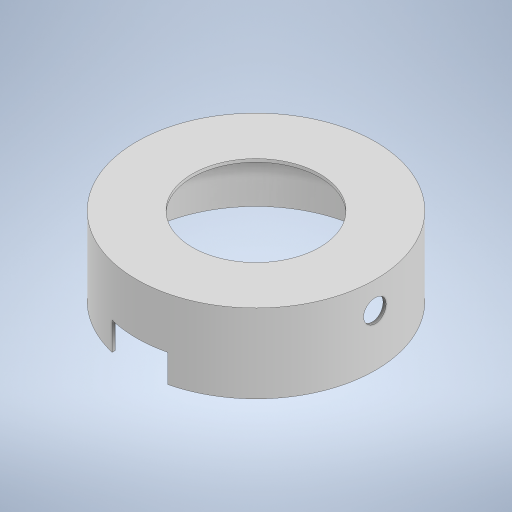
# Autodesk Inventor part: Diaphragm_lock
Saved by Autodesk Inventor 2023 (Build 270158000, 158)
## iProperties
Created: 2023-02-27
Part Number: Diaphragm_lock
Material: Generic
Document SubType Name: Modeling
Designer: maste
Density: 1 g/cm^3
Appearance: Default
Author: maste
Autodesk Inventor part; units mm, degrees
ref_plane "YZ Plane" through (0, 0, 0) normal (1, 0, 0) x (0, 1, 0)
ref_plane "XZ Plane" through (0, 0, 0) normal (0, 1, 0) x (-1, 0, 0)
ref_plane "XY Plane" through (0, 0, 0) normal (0, 0, 1) x (1, 0, 0)
sketch "Sketch1" plane through (0, 0, 0) normal (0, 0, 1) x (1, 0, 0)
  circle A0 centre (0, 0) radius 30
  dimension "d0" = 60
  constraints: 1 centre point, 1 coincident
  measures "d0" diameter of A0
extrude "Initial Cylinder" add sketch "Sketch1" along normal blind 4.78
sketch "Sketch2" plane through (0, 0, 4.78) normal (0, 0, 1) x (1, 0, 0)
  circle A0 centre (0, 0) radius 16
  dimension "d3" = 32
  constraints: 1 centre point, 1 coincident
  measures "d3" diameter of A0
extrude "Through-hole" cut sketch "Sketch2" against normal blind 548
sketch "Sketch3" plane through (0, 0, 4.78) normal (0, 0, 1) x (1, 0, 0)
  circle A0 centre (0, 0) radius 29.25
  dimension "d6" = 58.5
  constraints: 1 centre point, 1 coincident
  measures "d6" diameter of A0
extrude "snug ring fit" cut sketch "Sketch3" against normal blind 4
sketch "Sketch5" plane through (0, 0, 0) normal (0, 1, 0) x (-1, 0, 0)
  line L0 (30, 4.78) -> (-30, 4.78) projected
  line L1 (30, 0) -> (-30, 0) projected
  point P0 (0, 0)
  dimension "d16" = 4.78
  measures "d16" distance between parallel lines of L0 L1
sketch "Sketch6" plane through (0, 0, 0.78) normal (0, 0, 1) x (1, 0, 0)
  circle A0 centre (0, 0) radius 17.65
  dimension "d17" = 35.3
  constraints: 1 centre point, 1 coincident
  measures "d17" diameter of A0
extrude "Piezo Puzzle indent" cut sketch "Sketch6" against normal blind 0.5
sketch "Sketch7" plane through (0, 0, 0) normal (0, 0, -1) x (-1, 0, 0)
  circle A0 centre (0, 0) radius 16 projected
  circle A1 centre (0, 0) radius 30 projected
extrude "Extra forward thickness" add sketch "Sketch7" along normal blind 1
sketch "Sketch8" plane through (0, 0, 0.28) normal (0, 0, 1) x (1, 0, 0)
  circle A0 centre (0, 0) radius 16 projected
  circle A1 centre (0, 0) radius 17.65 projected
  circle A2 centre (0, 0) radius 17.75
  dimension "d26" = 35.5
  constraints: 1 centre point, 1 coincident
  measures "d26" diameter of A2
extrude "Piezo accomodation for EFT^" cut sketch "Sketch8" along normal mid plane 1 contours A0 | A1 | A2
sketch "Sketch9" plane through (0, 0, 4.78) normal (0, 0, 1) x (1, 0, 0)
  circle A0 centre (0, 0) radius 29.25 projected
  circle A1 centre (0, 0) radius 30 projected
extrude "Downoward extension" add sketch "Sketch9" along normal blind 14
sketch "Sketch4" plane through (0, 0, 0) normal (0, 1, 0) x (-1, 0, 0)
  line L0 (30, 4.78) -> (-30, 4.78) projected
  line L1 (0, 4.78) -> (0, 5.78)
  circle A0 centre (0, 5.78) radius 2.825
  point P0 (0, 0)
  dimension "d10" = 5.65
  dimension "d29" = 1
  constraints: 2 end point, 1 centre point, 1 coincident, 1 midpoint, 1 vertical
  measures "d10" diameter of A0
  measures "d29" distance of L1.start L1.end
extrude "Bolt through-hole" cut sketch "Sketch4" along normal mid plane 548
sketch "Sketch11" plane through (0, 0, 18.78) normal (0, 0, 1) x (1, 0, 0)
  line L0 (0, 0) -> (-30, 0)
  circle A0 centre (0, 0) radius 30 projected
  line L1 (-27.0677, -7) -> (-27.0677, 7)
  line L2 (-27.0677, 7) -> (-32.9323, 7)
  line L3 (-32.9323, 7) -> (-32.9323, -7)
  line L4 (-32.9323, -7) -> (-27.0677, -7)
  line L5 (-27.0677, -7) -> (-32.9323, 7) construction
  line L6 (-27.0677, 7) -> (-32.9323, -7) construction
  point P0 (-29.1719, 7)
  point P1 (-29.1719, -7)
  dimension "d32" = 14
  constraints: 14 end point, 2 midpoint, 2 parallel, 1 horizontal, 1 perpendicular, 1 vertical, 2 other
  measures "d32" distance of L1.start L1.end
extrude "Extrusion10" cut sketch "Sketch11" against normal blind 7 contours L1 L4 A0 L0 | L0 A0 L2 L1
body "Solid1"
